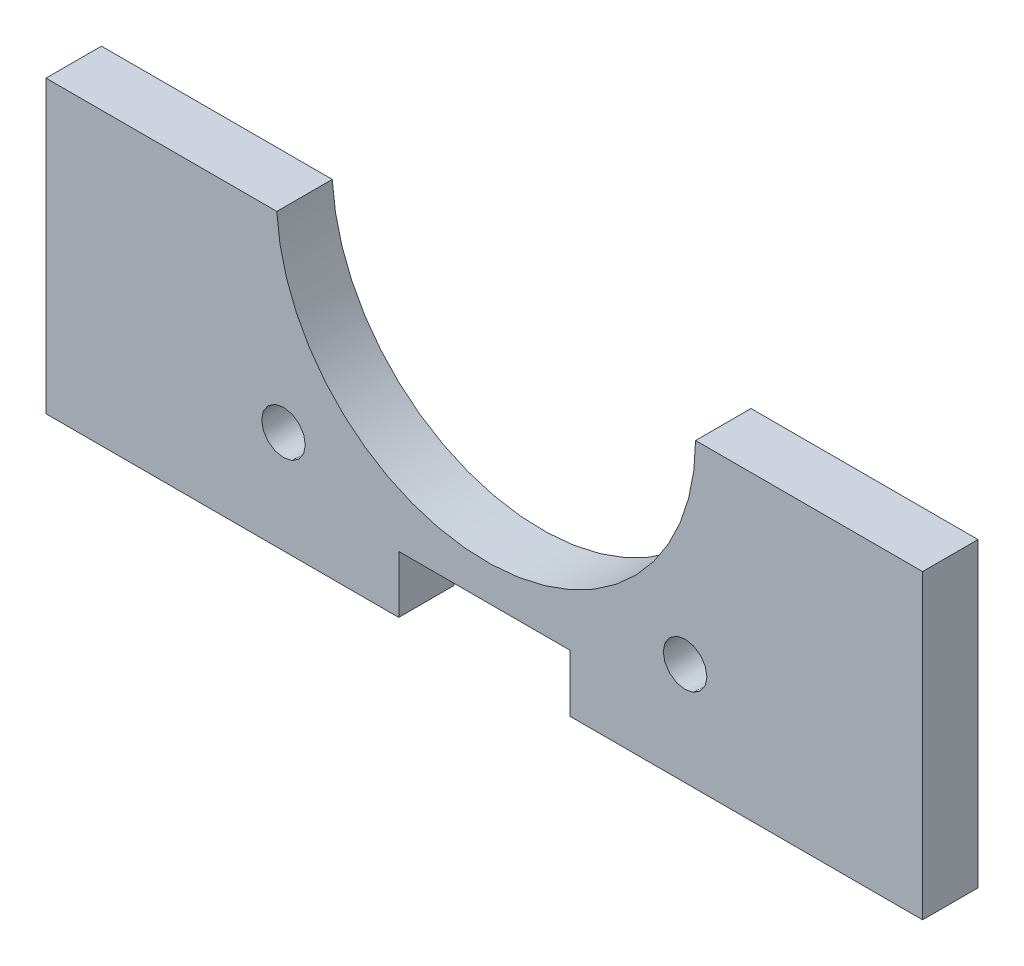
# Autodesk Inventor part: side_plate_bottom
Saved by Autodesk Inventor 2017 (Build 210142000, 142)
## iProperties
Created: 2017-06-15
Part Number: side_plate_bottom
Material: Generic
Document SubType Name: Modeling
Designer: millerid
Density: 1 g/cm^3
Appearance: Default
Author: millerid
Autodesk Inventor part; units mm, degrees
ref_plane "YZ Plane" through (0, 0, 0) normal (1, 0, 0) x (0, 1, 0)
ref_plane "XZ Plane" through (0, 0, 0) normal (0, 1, 0) x (-1, 0, 0)
ref_plane "XY Plane" through (0, 0, 0) normal (0, 0, 1) x (1, 0, 0)
sketch "Sketch1" plane through (0, 0, 0) normal (0, 0, 1) x (1, 0, 0)
  line L0 (20.2032, 0.2766) -> (20.2032, -3)
  line L1 (20.2032, -3) -> (0, -3)
  line L2 (0, -3) -> (0, 0)
  line L3 (30, 0.2766) -> (30, -3)
  line L4 (30, -3) -> (50.2032, -3)
  line L5 (50.2032, -3) -> (50.2032, 0)
  line L6 (20.2032, 0.2766) -> (30, 0.2766)
  circle A0 centre (13.6016, 2.8766) radius 1.25
  circle A1 centre (36.6016, 2.8766) radius 1.25
  arc A2 (13.2197, 13.6484) -> (37.2032, 14.2766) centre (25.2032, 14.2766) ccw
  line L7 (37.2032, 14.2766) -> (50.2032, 14.2766)
  line L8 (50.2032, 14.2766) -> (50.2032, 0)
  line L9 (13.2197, 13.6484) -> (0, 13.6484)
  line L10 (0, 13.6484) -> (0, 0)
  point P0 (25.1016, 0.2766)
  dimension "d2" = 20.2032
  dimension "d3" = 3.2766
  dimension "d4" = 20.2032
  dimension "d11" = 2.5
  dimension "d12" = 2.6
  dimension "d13" = 11.5
  dimension "d14" = 2.5
  dimension "d15" = 11.5
  dimension "d22" = 12
  dimension "d23" = 13.2196
  constraints: 22 end point, 3 centre point, 3 horizontal, 2 parallel, 2 perpendicular, 2 point on circle, 1 midpoint, 1 point on line
  measures "d2" distance of L0.end L1.end
  measures "d3" distance of L0.start L0.end
  measures "d4" distance of L4.end L3.end
  measures "d11" diameter of A0
  measures "d12" distance from line of L6 A0.centre
  measures "d13" horizontal distance of A0.centre point (25.102, 0.277)
  measures "d14" diameter of A1
  measures "d15" horizontal distance of A1.centre point (25.102, 0.277)
  measures "d22" radius of A2
  measures "d23" distance of L9.start L9.end
extrude "Extrusion2" add sketch "Sketch1" along normal blind 3.175
equation "\"d4\" = d2"
equation "\"d15\" = d13"
body "Solid2"
